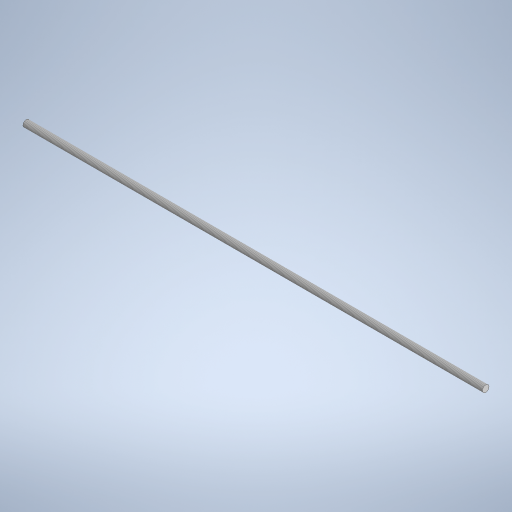
# Autodesk Inventor part: shaftdrive
Saved by Autodesk Inventor 2024 (Build 280153000, 153)
## iProperties
Created: 2023-12-14
Part Number: shaftdrive
Material: Generic
Document SubType Name: Modeling
Designer: Abdulrahman Riskuwa
Density: 1 g/cm^3
Appearance: Default
Author: Abdulrahman Riskuwa
Autodesk Inventor part; units mm, degrees
ref_plane "YZ Plane" through (0, 0, 0) normal (1, 0, 0) x (0, 1, 0)
ref_plane "XZ Plane" through (0, 0, 0) normal (0, 1, 0) x (-1, 0, 0)
ref_plane "XY Plane" through (0, 0, 0) normal (0, 0, 1) x (1, 0, 0)
sketch "Sketch1" plane through (0, 0, 0) normal (1, 0, 0) x (0, 1, 0)
  circle A0 centre (0, 0) radius 1.8
  dimension "d0" = 3.6
  constraints: 1 centre point, 1 coincident
  measures "d0" diameter of A0
extrude "Extrusion1" add sketch "Sketch1" along normal blind 252
thread "Thread1" size "M3.5x0.6" class "6g" standard "ISO Metric profile" full length
body "Solid1"
